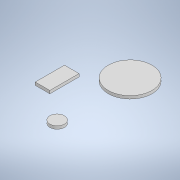
# Autodesk Inventor part: multi
Saved by Autodesk Inventor 2020.2 (Build 242310000, 310)
## iProperties
Created: 2021-04-26
Part Number: multi
Material: Generic
Document SubType Name: Modeling
Designer: Tarsoly
Density: 1 g/cm^3
Appearance: Default
Author: Tarsoly
Autodesk Inventor part; units mm, degrees
ref_plane "YZ Plane" through (0, 0, 0) normal (1, 0, 0) x (0, 1, 0)
ref_plane "XZ Plane" through (0, 0, 0) normal (0, 1, 0) x (-1, 0, 0)
ref_plane "XY Plane" through (0, 0, 0) normal (0, 0, 1) x (1, 0, 0)
sketch "Sketch1" plane through (0, 0, 0) normal (0, 1, 0) x (-1, 0, 0)
  line L0 (2500, 2500) -> (-2500, 2500)
  line L1 (-2500, 2500) -> (-2500, -2500)
  line L2 (-2500, -2500) -> (2500, -2500)
  line L3 (2500, -2500) -> (2500, 2500)
  line L4 (2500, 2500) -> (-2500, -2500) construction
  line L5 (-2500, 2500) -> (2500, -2500) construction
  line L6 (2500, 0) -> (-2500, 0) construction
  line L7 (0, 2500) -> (0, -2500) construction
  circle A0 centre (0, 1250) radius 250
  circle A1 centre (0, -1250) radius 750
  line L8 (1000, -500) -> (1500, -500)
  line L9 (1500, -500) -> (1500, 500)
  line L10 (1500, 500) -> (1000, 500)
  line L11 (1000, 500) -> (1000, -500)
  line L12 (1000, -500) -> (1500, 500)
  line L13 (1500, -500) -> (1000, 500)
  point P0 (0, 0)
  point P1 (1250, 0)
  dimension "d0" = 5000
  dimension "d1" = 5000
  dimension "d2" = 500
  dimension "d3" = 1500
  dimension "d4" = 500
  dimension "d5" = 1000
  constraints: 28 end point, 8 midpoint, 4 parallel, 2 centre point, 2 horizontal, 2 perpendicular, 1 point on line
  measures "d0" distance of L2.end L1.end
  measures "d1" distance of L1.end L0.end
  measures "d2" diameter of A0
  measures "d3" diameter of A1
  measures "d4" distance of L10.end L9.end
  measures "d5" distance of L9.end L8.end
extrude "Extrusion1" add sketch "Sketch1" along normal blind 100 contours A0 | A1 | L12 L13 L8 | L11 L13 L12 | L13 L12 L9 | L10 L12 L13
body "Solid1"
